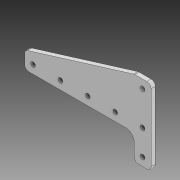
# Autodesk Inventor part: Cart Carrier
Saved by Autodesk Inventor 2020 (Build 240168000, 168)
## iProperties
Created: 2020-10-19
Part Number: Cart Carrier
Material: Generic
Document SubType Name: Modeling
Designer: DDeGo
Density: 1 g/cm^3
Appearance: Default
Author: DDeGo
Autodesk Inventor part; units mm, degrees
ref_plane "YZ Plane" through (0, 0, 0) normal (1, 0, 0) x (0, 1, 0)
ref_plane "XZ Plane" through (0, 0, 0) normal (0, 1, 0) x (-1, 0, 0)
ref_plane "XY Plane" through (0, 0, 0) normal (0, 0, 1) x (1, 0, 0)
sketch "Sketch1" plane through (0, 0, 0) normal (0, 0, 1) x (1, 0, 0)
  line L0 (-75, -10) -> (55, -10)
  line L1 (75, -10) -> (75, 10)
  line L2 (75, 10) -> (-75, 10) construction
  line L3 (-75, 10) -> (-75, -10)
  line L4 (-75, -10) -> (75, 10) construction
  line L5 (75, -10) -> (-75, 10) construction
  line L6 (75, 10) -> (75, 50)
  line L7 (75, 50) -> (55, 50)
  line L8 (75, -40) -> (75, -10)
  line L9 (-65, 10) -> (-65, -10) construction
  line L10 (55, -40) -> (75, -40)
  line L11 (55, -40) -> (55, -10)
  line L12 (65, 50) -> (65, -40) construction
  line L13 (-65, 0) -> (0, 0) construction
  line L14 (0, 0) -> (65, 5) construction
  circle A0 centre (-65, 0) radius 2.75
  circle A1 centre (65, 40) radius 2.75
  circle A2 centre (65, -30) radius 2.75
  line L15 (55, -10) -> (55, 50) construction
  line L16 (55, -10) -> (75, -10) construction
  line L17 (-75, 10) -> (55, 50)
  dimension "d8" = 20
  dimension "d9" = 130
  dimension "d13" = 10
  dimension "d14" = 10
  dimension "d15" = 5.5
  dimension "d16" = 10
  dimension "d17" = 10
  dimension "d18" = 10
  dimension "d22" = 40
  dimension "d23" = 30
  constraints: 36 end point, 7 perpendicular, 6 midpoint, 4 horizontal, 4 point on line, 4 vertical, 3 centre point, 3 parallel, 2 equal radius, 1 coincident
  measures "d8" distance of L1.start L1.end
  measures "d9" distance between parallel lines of L12 L9
  measures "d13" distance from line of L10 A2.centre
  measures "d14" distance from line of L7 A1.centre
  measures "d15" diameter of A2
  measures "d16" distance between parallel lines of L8 L12
  measures "d17" distance between parallel lines of L11 L12
  measures "d18" distance between parallel lines of L3 L9
  measures "d22" distance of L1.end L6.end
  measures "d23" distance of L8.start L1.start
extrude "Extrusion1" add sketch "Sketch1" along normal blind 5
fillet "Fillet1" radius 10 1 edges at (55, -10, 2.5)
fillet "Fillet1" radius 5 6 edges at (55, -40, 2.5) (75, -40, 2.5) (-75, -10, 2.5) (-75, 10, 2.5) (55, 50, 2.5) (75, 50, 2.5)
sketch "Sketch3" plane through (0, 0, 0) normal (0, 0, -1) x (-1, 0, 0)
  circle A0 centre (0, 0) radius 2.75
  line L0 (70, -10) -> (-45, -10) projected
  line L1 (0, 0) -> (-32.5, 0) construction
  line L2 (0, 0) -> (32.5, 0) construction
  circle A1 centre (-32.5, 0) radius 2.75
  circle A2 centre (32.5, 0) radius 2.75
  line L3 (-32.5, 0) -> (-65, 0) construction
  circle A3 centre (-65, 0) radius 2.75
  dimension "d24" = 5.5
  dimension "d28" = 32.5
  constraints: 6 end point, 4 centre point, 4 coincident, 3 equal radius, 3 horizontal, 2 collinear
  measures "d24" diameter of A0
  measures "d28" distance of L1.start L1.end
extrude "Extrusion3" cut sketch "Sketch3" against normal through all
equation "\"d14\" = d13"
body "Solid1"
